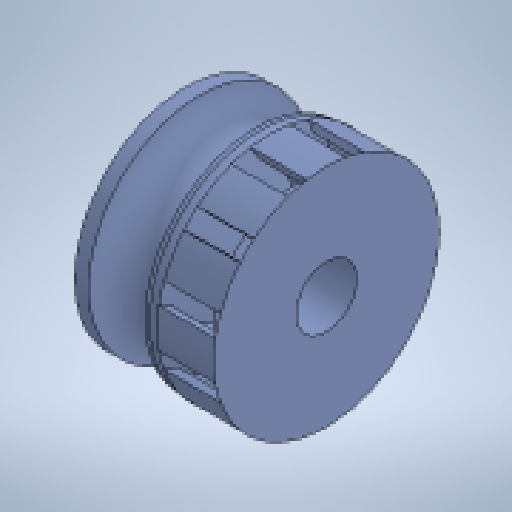
# Autodesk Inventor part: Idler - Puley
Saved by Autodesk Inventor 2023.2 (Build 272271000, 271)
## iProperties
Created: 2023-11-16
Part Number: Idler - Puley
Material: Nylon 6/6
Document SubType Name: Modeling
Designer: Nathan Cai
Density: 1.13 g/cm^3
Appearance: Rubber - Blue
Author: Nathan Cai
Autodesk Inventor part; units mm, degrees
ref_plane "YZ Plane" through (0, 0, 0) normal (1, 0, 0) x (0, 1, 0)
ref_plane "XZ Plane" through (0, 0, 0) normal (0, 1, 0) x (-1, 0, 0)
ref_plane "XY Plane" through (0, 0, 0) normal (0, 0, 1) x (1, 0, 0)
sketch "Sketch1" plane through (0, 0, 0) normal (0, 0, 1) x (1, 0, 0)
  line L0 (-4.7625, -12.5) -> (4.7625, -12.5)
  line L1 (4.7625, -12.5) -> (4.7625, 12.5)
  line L2 (4.7625, 12.5) -> (-4.7625, 12.5)
  line L3 (-4.7625, 12.5) -> (-4.7625, -12.5)
  line L4 (-4.7625, -12.5) -> (4.7625, 12.5) construction
  line L5 (4.7625, -12.5) -> (-4.7625, 12.5) construction
  circle A0 centre (0, 12.5) radius 3.175
  line L6 (-4.7625, -3.429) -> (4.7625, -3.429)
  line L7 (4.7625, -3.429) -> (4.7625, 3.429)
  line L8 (4.7625, 3.429) -> (-4.7625, 3.429)
  line L9 (-4.7625, 3.429) -> (-4.7625, -3.429)
  line L10 (-4.7625, -3.429) -> (4.7625, 3.429) construction
  line L11 (4.7625, -3.429) -> (-4.7625, 3.429) construction
  line L12 (-4.7625, 0) -> (4.7625, 0) construction
  point P0 (0, 0)
  point P1 (3.175, 12.5)
  point P2 (-3.175, 12.5)
  dimension "d0" = 9.525
  dimension "d1" = 25
  dimension "d2" = 6.35
  dimension "d3" = 9.525
  dimension "d4" = 6.858
  constraints: 26 end point, 7 midpoint, 4 parallel, 2 horizontal, 2 perpendicular, 1 centre point
  measures "d0" distance of L2.end L1.end
  measures "d1" distance of L1.end L0.end
  measures "d2" diameter of A0
  measures "d3" distance of L8.end L7.end
  measures "d4" distance of L7.end L6.end
revolve "Revolution1" add sketch "Sketch1" angle 360 about axis through (-4.7625, 0, 0) along (1, 0, 0) contours L3 L2 A0 L1 L8
sketch "Sketch3" plane through (0, 0, 0) normal (0, 1, 0) x (-1, 0, 0)
  line L0 (-4.7625, 12.5) -> (-4.7625, -12.5) projected
  line L1 (-4.7625, 12.7) -> (-11.1125, 12.7)
  line L2 (-11.1125, 12.7) -> (-11.1125, -12.7)
  line L3 (-11.1125, -12.7) -> (-4.7625, -12.7) construction
  line L4 (-4.7625, -12.7) -> (-4.7625, 12.7)
  line L5 (-4.7625, 12.7) -> (-11.1125, -12.7) construction
  line L6 (-11.1125, 12.7) -> (-4.7625, -12.7) construction
  line L7 (4.7625, 12.5) -> (4.7625, -12.5) projected
  line L8 (4.7625, 0) -> (-4.7625, 0) construction
  line L9 (-7.9375, -12.7) -> (-7.9375, 12.7) construction
  line L10 (-4.7625, -12.7) -> (-7.9375, -9.525)
  line L11 (-11.1125, -12.7) -> (-7.9375, -9.525)
  line L12 (-11.1125, 3.429) -> (-4.7625, 3.429)
  line L13 (-4.7625, 3.429) -> (-4.7625, -3.429)
  line L14 (-4.7625, -3.429) -> (-11.1125, -3.429)
  line L15 (-11.1125, -3.429) -> (-11.1125, 3.429)
  line L16 (-11.1125, 3.429) -> (-4.7625, -3.429) construction
  line L17 (-4.7625, 3.429) -> (-11.1125, -3.429) construction
  point P0 (0, 0)
  point P1 (-7.9375, 0)
  point P2 (-4.7625, -3.429)
  dimension "d14" = 6.35
  dimension "d15" = 25.4
  dimension "d16" = 6.35
  dimension "d17" = 6.858
  constraints: 32 end point, 8 midpoint, 4 parallel, 4 perpendicular, 3 point on line, 2 horizontal
  measures "d14" distance of L3.end L2.end
  measures "d15" distance of L2.end L1.end
  measures "d16" distance of L13.end L14.end
  measures "d17" distance of L12.end L13.end
revolve "Revolution2" add sketch "Sketch3" angle 360 about axis through (-4.7625, 0, 0) along (1, 0, 0) contours L0 L4 L10 L11 L2 L14
fillet "Fillet1" radius 3.175 1 edges at (4.7625, -12.5, 0)
sketch "Sketch4" plane through (11.1125, 0, 0) normal (1, 0, 0) x (0, 0, -1)
  circle A0 centre (0, 0) radius 12.7 projected
  circle A1 centre (0, 0) radius 3.429 projected
  arc A2 (11.7254, -2.0675) -> (11.7254, 2.0675) centre (0, 0) ccw
  circle A3 centre (0, 0) radius 9.525
  line L0 (9.5064, 0.5953) -> (11.8914, 0.5953)
  line L1 (11.8914, 0.5953) -> (11.8914, -0.5953) construction
  line L2 (11.8914, -0.5953) -> (9.5064, -0.5953)
  line L3 (9.5064, -0.5953) -> (9.5064, 0.5953) construction
  line L4 (9.5064, 0.5953) -> (11.8914, -0.5953) construction
  line L5 (11.8914, 0.5953) -> (9.5064, -0.5953) construction
  circle A4 centre (0, 0) radius 12.7 projected
  line L6 (12.7, 0) -> (0, 0) construction
  circle A5 centre (0, 0) radius 3.429 projected
  line L7 (0, 0) -> (12.5071, -2.2053) construction
  line L8 (11.7254, -2.0675) -> (12.5071, -2.2053)
  line L9 (11.7254, 2.0675) -> (12.5071, 2.2053)
  line L10 (8.5304, 4.2376) -> (7.9351, 5.2687) construction
  line L11 (7.9351, 5.2687) -> (10.0006, 6.4612)
  line L12 (10.5959, 5.4301) -> (8.5304, 4.2376)
  line L13 (7.9351, 5.2687) -> (10.5959, 5.4301) construction
  line L14 (10.0006, 6.4612) -> (8.5304, 4.2376) construction
  line L15 (10.0006, 6.4612) -> (10.5959, 5.4301) construction
  arc A6 (11.1882, 4.0722) -> (9.1207, 7.6532) centre (0, 0) ccw
  line L16 (11.1882, 4.0722) -> (11.9341, 4.3437)
  line L17 (9.1207, 7.6532) -> (9.7288, 8.1634)
  line L18 (5.2687, 7.9351) -> (4.2376, 8.5304) construction
  line L19 (4.2376, 8.5304) -> (5.4301, 10.5959)
  line L20 (6.4612, 10.0006) -> (5.2687, 7.9351)
  line L21 (4.2376, 8.5304) -> (6.4612, 10.0006) construction
  line L22 (5.4301, 10.5959) -> (5.2687, 7.9351) construction
  line L23 (5.4301, 10.5959) -> (6.4612, 10.0006) construction
  arc A7 (7.6532, 9.1207) -> (4.0722, 11.1882) centre (0, 0) ccw
  line L24 (7.6532, 9.1207) -> (8.1634, 9.7288)
  line L25 (4.0722, 11.1882) -> (4.3437, 11.9341)
  line L26 (0.5953, 9.5064) -> (-0.5953, 9.5064) construction
  line L27 (-0.5953, 9.5064) -> (-0.5953, 11.8914)
  line L28 (0.5953, 11.8914) -> (0.5953, 9.5064)
  line L29 (-0.5953, 9.5064) -> (0.5953, 11.8914) construction
  line L30 (-0.5953, 11.8914) -> (0.5953, 9.5064) construction
  line L31 (-0.5953, 11.8914) -> (0.5953, 11.8914) construction
  arc A8 (2.0675, 11.7254) -> (-2.0675, 11.7254) centre (0, 0) ccw
  line L32 (2.0675, 11.7254) -> (2.2053, 12.5071)
  line L33 (-2.0675, 11.7254) -> (-2.2053, 12.5071)
  line L34 (-4.2376, 8.5304) -> (-5.2687, 7.9351) construction
  line L35 (-5.2687, 7.9351) -> (-6.4612, 10.0006)
  line L36 (-5.4301, 10.5959) -> (-4.2376, 8.5304)
  line L37 (-5.2687, 7.9351) -> (-5.4301, 10.5959) construction
  line L38 (-6.4612, 10.0006) -> (-4.2376, 8.5304) construction
  line L39 (-6.4612, 10.0006) -> (-5.4301, 10.5959) construction
  arc A9 (-4.0722, 11.1882) -> (-7.6532, 9.1207) centre (0, 0) ccw
  line L40 (-4.0722, 11.1882) -> (-4.3437, 11.9341)
  line L41 (-7.6532, 9.1207) -> (-8.1634, 9.7288)
  line L42 (-7.9351, 5.2687) -> (-8.5304, 4.2376) construction
  line L43 (-8.5304, 4.2376) -> (-10.5959, 5.4301)
  line L44 (-10.0006, 6.4612) -> (-7.9351, 5.2687)
  line L45 (-8.5304, 4.2376) -> (-10.0006, 6.4612) construction
  line L46 (-10.5959, 5.4301) -> (-7.9351, 5.2687) construction
  line L47 (-10.5959, 5.4301) -> (-10.0006, 6.4612) construction
  arc A10 (-9.1207, 7.6532) -> (-11.1882, 4.0722) centre (0, 0) ccw
  line L48 (-9.1207, 7.6532) -> (-9.7288, 8.1634)
  line L49 (-11.1882, 4.0722) -> (-11.9341, 4.3437)
  line L50 (-9.5064, 0.5953) -> (-9.5064, -0.5953) construction
  line L51 (-9.5064, -0.5953) -> (-11.8914, -0.5953)
  line L52 (-11.8914, 0.5953) -> (-9.5064, 0.5953)
  line L53 (-9.5064, -0.5953) -> (-11.8914, 0.5953) construction
  line L54 (-11.8914, -0.5953) -> (-9.5064, 0.5953) construction
  line L55 (-11.8914, -0.5953) -> (-11.8914, 0.5953) construction
  arc A11 (-11.7254, 2.0675) -> (-11.7254, -2.0675) centre (0, 0) ccw
  line L56 (-11.7254, 2.0675) -> (-12.5071, 2.2053)
  line L57 (-11.7254, -2.0675) -> (-12.5071, -2.2053)
  line L58 (-8.5304, -4.2376) -> (-7.9351, -5.2687) construction
  line L59 (-7.9351, -5.2687) -> (-10.0006, -6.4612)
  line L60 (-10.5959, -5.4301) -> (-8.5304, -4.2376)
  line L61 (-7.9351, -5.2687) -> (-10.5959, -5.4301) construction
  line L62 (-10.0006, -6.4612) -> (-8.5304, -4.2376) construction
  line L63 (-10.0006, -6.4612) -> (-10.5959, -5.4301) construction
  arc A12 (-11.1882, -4.0722) -> (-9.1207, -7.6532) centre (0, 0) ccw
  line L64 (-11.1882, -4.0722) -> (-11.9341, -4.3437)
  line L65 (-9.1207, -7.6532) -> (-9.7288, -8.1634)
  line L66 (-5.2687, -7.9351) -> (-4.2376, -8.5304) construction
  line L67 (-4.2376, -8.5304) -> (-5.4301, -10.5959)
  line L68 (-6.4612, -10.0006) -> (-5.2687, -7.9351)
  line L69 (-4.2376, -8.5304) -> (-6.4612, -10.0006) construction
  line L70 (-5.4301, -10.5959) -> (-5.2687, -7.9351) construction
  line L71 (-5.4301, -10.5959) -> (-6.4612, -10.0006) construction
  arc A13 (-7.6532, -9.1207) -> (-4.0722, -11.1882) centre (0, 0) ccw
  line L72 (-7.6532, -9.1207) -> (-8.1634, -9.7288)
  line L73 (-4.0722, -11.1882) -> (-4.3437, -11.9341)
  line L74 (-0.5953, -9.5064) -> (0.5953, -9.5064) construction
  line L75 (0.5953, -9.5064) -> (0.5953, -11.8914)
  line L76 (-0.5953, -11.8914) -> (-0.5953, -9.5064)
  line L77 (0.5953, -9.5064) -> (-0.5953, -11.8914) construction
  line L78 (0.5953, -11.8914) -> (-0.5953, -9.5064) construction
  line L79 (0.5953, -11.8914) -> (-0.5953, -11.8914) construction
  arc A14 (-2.0675, -11.7254) -> (2.0675, -11.7254) centre (0, 0) ccw
  line L80 (-2.0675, -11.7254) -> (-2.2053, -12.5071)
  line L81 (2.0675, -11.7254) -> (2.2053, -12.5071)
  line L82 (4.2376, -8.5304) -> (5.2687, -7.9351) construction
  line L83 (5.2687, -7.9351) -> (6.4612, -10.0006)
  line L84 (5.4301, -10.5959) -> (4.2376, -8.5304)
  line L85 (5.2687, -7.9351) -> (5.4301, -10.5959) construction
  line L86 (6.4612, -10.0006) -> (4.2376, -8.5304) construction
  line L87 (6.4612, -10.0006) -> (5.4301, -10.5959) construction
  arc A15 (4.0722, -11.1882) -> (7.6532, -9.1207) centre (0, 0) ccw
  line L88 (4.0722, -11.1882) -> (4.3437, -11.9341)
  line L89 (7.6532, -9.1207) -> (8.1634, -9.7288)
  line L90 (7.9351, -5.2687) -> (8.5304, -4.2376) construction
  line L91 (8.5304, -4.2376) -> (10.5959, -5.4301)
  line L92 (10.0006, -6.4612) -> (7.9351, -5.2687)
  line L93 (8.5304, -4.2376) -> (10.0006, -6.4612) construction
  line L94 (10.5959, -5.4301) -> (7.9351, -5.2687) construction
  line L95 (10.5959, -5.4301) -> (10.0006, -6.4612) construction
  arc A16 (9.1207, -7.6532) -> (11.1882, -4.0722) centre (0, 0) ccw
  line L96 (9.1207, -7.6532) -> (9.7288, -8.1634)
  line L97 (11.1882, -4.0722) -> (11.9341, -4.3437)
  point P0 (10.6989, 0)
  point P1 (9.2655, 5.3494)
  point P2 (10.9985, 6.35)
  point P3 (5.3494, 9.2655)
  point P4 (6.35, 10.9985)
  point P5 (0, 10.6989)
  point P6 (0, 12.7)
  point P7 (-5.3494, 9.2655)
  point P8 (-6.35, 10.9985)
  point P9 (-9.2655, 5.3494)
  point P10 (-10.9985, 6.35)
  point P11 (-10.6989, 0)
  point P12 (-12.7, 0)
  point P13 (-9.2655, -5.3494)
  point P14 (-10.9985, -6.35)
  point P15 (-5.3494, -9.2655)
  point P16 (-6.35, -10.9985)
  point P17 (0, -10.6989)
  point P18 (0, -12.7)
  point P19 (5.3494, -9.2655)
  point P20 (6.35, -10.9985)
  point P21 (9.2655, -5.3494)
  point P22 (10.9985, -6.35)
  dimension "d21" = 19.05
  dimension "d20" = 0.7937
  dimension "d22" = 1.1906
  dimension "d23" = 10
  dimension "d26" = 360
  constraints: 196 end point, 38 point on circle, 12 centre point, 2 horizontal, 2 midpoint, 2 parallel, 2 point on line, 2 symmetric about line, 1 coincident, 1 collinear, 1 perpendicular, 245 other
  measures "d22" distance between parallel lines of L2 L0
  measures "d23" angle of L6 L7
extrude "Extrusion2" add sketch "Sketch4" against normal blind 6.35 contours A0 L8 A2 L9 | L16 A6 L17 A0 | A0 L96 A16 L97 | A2 L2 A3 L0 | L24 A7 L25 A0 | L12 A3 L11 A6 | A3 | A0 L88 A15 L89 | A16 L92 A3 L91 | L32 A8 L33 A0 | L20 A3 L19 A7 | A0 L80 A14 L81 | A15 L84 A3 L83 | L40 A9 L41 A0 | L28 A3 L27 A8 | A0 L72 A13 L73 | A14 L76 A3 L75 | L48 A10 L49 A0 | L36 A3 L35 A9 | A0 L64 A12 L65 | A13 L68 A3 L67 | L56 A11 L57 A0 | L44 A3 L43 A10 | A12 L60 A3 L59 | L52 A3 L51 A11
body "Solid1"
